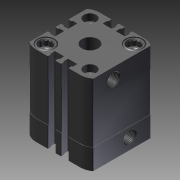
# Autodesk Inventor part: 536267 ADN-15-P---(Z)
Saved by Autodesk Inventor 2011 SP1 (Build 150282100, 282)
## iProperties
Created: 2018-05-26
Part Number: 536267 ADN-15-P---(Z)
Catalog Web Link: www.cadenas.de
Description: ADN-(Z)-Compact cylinder - Z
Vendor: FESTO
Document SubType Name: Modeling
Designer: psAdmin
Manufacturer: FESTO
Mass: 85.3695 g
Surface Area: 308.359 cm^2
Volume: 85.3695 cm^3
Density: 1 g/cm^3
Category: PARTsolutions
Company: FESTO
Title: 536267 ADN-15-P---(Z)
Author: Cadenas PARTsolutions
Comments: Compact cylinder - Z
PSOL_IDENT_0: {$CADENAS_DATA\23d-libs\festo\parts\a\adn\parts\adn_zr.prj},210 {VTYP=3D},{NB=536267 ADN-15-P---(Z)}
PSOL_IDENT_1: ,{LINA=536267 ADN-15-P---(Z)},{NN=ADN-(Z)},{DATE=06.10.2015 11:54:02},{GEOMDATE=22.09.2015 09:31:00}
PSOL_IDENT_2: ,{VERSION=},{LINEID=8220},{LINESUBID=-1},{WBVAR=HUB,DF,Q,S2S20,S1,R8,TT}  {NB=536267 ADN-15-P---(Z)}
PSOL_IDENT_3: ,{LINA=536267 ADN-15-P---(Z)},{KT=536267},{TNR=536267},{AUSF=ADN},{KDM=32},{BG=26.000},{VERS=2},{HUB
PSOL_IDENT_4: P=-},{HUB=15.00000},{HUB1=[1-400]},{HUB2=[1-300]},{HUB3=0},{THC='A','I'},{DF=P},{GA=A},{HUBL=variabl
PSOL_IDENT_5: e},{HUBC=hubc error},{Q=-},{VAR1C='-','Q'},{S2S20=-},{VAR2C='-','S2','S20'},{VAR5C='-','S6'},{S1=-},
PSOL_IDENT_6: {R8=-},{R81='-','R8'},{TT=-},{TT1='-','TT'},{VAR6C='-'},{VAR7C='-','R3'},{HUBALG=[1-400]},{A=19.000}
PSOL_IDENT_7: ,{A1=0.000},{AF=16.000},{AF1=0.000},{AF2=14.000},{AF3=0.000},{B=0.000},{B1=27.000},{BG1=0.000},{D1=9
PSOL_IDENT_8: .000},{D2=9.000},{D3=5.100},{D4=17.000},{D5=8.000},{D6=M5},{D7=5.000},{D8=4.500},{D9=8.000},{E=47.00
PSOL_IDENT_9: 0},{EE=G1/8},{EEN=9.728},{EE1=-},{J=15.000},{J1=6.000},{J11=6},{J2=0.000},{KF=5/16-24 UNF-2B},{KF1=-
PSOL_IDENT_10: },{KF2=10-32 UNF-2B},{KF3=-},{KK=3/8-24 UNF-2A},{KK1=-},{L1=3.300},{L2=44.000},{L3=2.100},{L4=5.000}
PSOL_IDENT_11: ,{L5=6.000},{L6=60.000},{L7=28.000},{L8=3.000},{L9=2.600},{L10=0.000},{L11=0.000},{MF=10.000},{MM=12
PSOL_IDENT_12: .000},{MM1=0.000},{PL=8.200},{RT=M6},{RTN=6},{RTNK=4.917},{SF=3/8},{SF1=-},{SW=10.000},{TG=32.500},{
PSOL_IDENT_13: VD=0.000},{VD1=6.400},{WH=6.200},{WH1=0.000},{WL=4.700},{WL1=0.000},{Y1=0.300},{Y2=0.500},{ZJ=50.200
PSOL_IDENT_14: },{ZM=56.400},{RU=35.200},{R1=12.400},{R2=1.000},{RA=9.700},{RB1=5.400},{RB2=6.800},{RT1=3.400},{DSK=
PSOL_IDENT_15: 9.000},{MDK=13.000},{MK=8.000},{MT=4.000},{MS=6.000},{RUB=0.600},{KFN=8.000},{KFK=6.647},{B111=12.80
PSOL_IDENT_16: 0},{B11=1.000},{B2=7.000},{B3=11.900},{B4=4.600},{B5=4.400},{B6=8.500},{B7=26.000},{B8=6.000},{B9=9.
PSOL_IDENT_17: 000},{B10=10.000},{W=0.400},{S=8.000},{LA=0.000},{LA1=0.000},{LA2=8.000},{LA3=12.500},{LA31=12.500},
PSOL_IDENT_18: {LA4=0.000},{LA5=0.000},{LA6=0.000},{RR=6.000},{LA7=0.000},{LA8=0.000},{LA9=0.000},{LA10=0.000},{ES=
PSOL_IDENT_19: 0.000},{SS=0.000},{TS=0.000},{WS=0.000},{DK=0.000},{KS=0.000},{QN=},{S2N=},{S1S20N=},{R8N=},{TTN=},{
PSOL_IDENT_20: DFALG='P','PPS'}
NN: ADN-(Z)
NT: Compact cylinder - Z
NB: 536267 ADN-15-P---(Z)
NBSYN: $TNR. $AUSF.-$HUB.-$DF.$QN.$S2N.$S1S20N.$R8N.$TTN.---(Z)
LINA: 536267 ADN-15-P---(Z)
TNR: 536267
AUSF: ADN
KDM: 32
BG: 26.000
HUB: 15.00000
DF: P
GA: A
Q: -
S2S20: -
S1: -
R8: -
TT: -
A: 19.000
A1: 0.000
AF: 16.000
AF1: 0.000
AF2: 14.000
AF3: 0.000
B: 0.000
B1: 27.000
BG1: 0.000
D1: 9.000
D2: 9.000
D3: 5.100
D4: 17.000
D5: 8.000
D6: M5
D7: 5.000
D8: 4.500
D9: 8.000
E: 47.000
EE: G1/8
EE1: -
J: 15.000
J1: 6.000
J2: 0.000
KF: 5/16-24 UNF-2B
KF1: -
KF2: 10-32 UNF-2B
KF3: -
KK: 3/8-24 UNF-2A
KK1: -
L1: 3.300
L2: 44.000
L3: 2.100
L4: 5.000
L5: 6.000
L6: 60.000
L7: 28.000
L8: 3.000
L9: 2.600
L10: 0.000
L11: 0.000
MF: 10.000
MM: 12.000
MM1: 0.000
PL: 8.200
RT: M6
RTNK: 4.917
SF: 3/8
SF1: -
SW: 10.000
TG: 32.500
VD: 0.000
VD1: 6.400
WH: 6.200
WH1: 0.000
WL: 4.700
WL1: 0.000
Y1: 0.300
Y2: 0.500
ZJ: 50.200
ZM: 56.400
RU: 35.200
R1: 12.400
R2: 1.000
RA: 9.700
DSK: 9.000
MDK: 13.000
MK: 8.000
MT: 4.000
MS: 6.000
RUB: 0.600
B111: 12.800
B11: 1.000
B2: 7.000
B3: 11.900
B4: 4.600
B5: 4.400
B6: 8.500
B7: 26.000
B8: 6.000
B9: 9.000
B10: 10.000
W: 0.400
S: 8.000
LA: 0.000
LA1: 0.000
LA2: 8.000
LA3: 12.500
LA31: 12.500
LA4: 0.000
LA5: 0.000
LA6: 0.000
RR: 6.000
LA7: 0.000
LA8: 0.000
LA9: 0.000
LA10: 0.000
ES: 0.000
SS: 0.000
TS: 0.000
WS: 0.000
DK: 0.000
KS: 0.000
SUPPLIER: FESTO
ARTICLENO: 536267 ADN-15-P---(Z)
BOMINFO: 536267 ADN-15-P---(Z)
CREATOR: CADENAS GmbH
Autodesk Inventor part; units mm, degrees
sketch "Skizze_2" plane through (0, 0, 0) normal (0, 0, 1) x (1, 0, 0)
  arc A0 (-23.5, -1.75) -> (-23.1, -2.15) centre (-23.1, -1.75) ccw
  line L0 (-23.1, -2.15) -> (-21.2, -2.15)
  arc A1 (-21.2, -2.15) -> (-21, -1.95) centre (-21.2, -1.95) ccw
  line L1 (-21, -1.95) -> (-21, -1.65)
  arc A2 (-20.8, -1.45) -> (-21, -1.65) centre (-20.8, -1.65) ccw
  line L2 (-20.8, -1.45) -> (-18, -1.45)
  arc A3 (-17.6, -1.85) -> (-18, -1.45) centre (-18, -1.85) ccw
  line L3 (-17.6, -1.85) -> (-17.6, -7.85)
  arc A4 (-18, -8.25) -> (-17.6, -7.85) centre (-18, -7.85) ccw
  line L4 (-18, -8.25) -> (-20.8, -8.25)
  arc A5 (-21, -8.05) -> (-20.8, -8.25) centre (-20.8, -8.05) ccw
  line L5 (-21, -8.05) -> (-21, -7.75)
  arc A6 (-21, -7.75) -> (-21.2, -7.55) centre (-21.2, -7.75) ccw
  line L6 (-21.2, -7.55) -> (-23.1, -7.55)
  arc A7 (-23.1, -7.55) -> (-23.5, -7.95) centre (-23.1, -7.95) ccw
  line L7 (-23.5, -7.95) -> (-23.5, -20.634)
  arc A8 (-23.5, -20.634) -> (-23.0482, -21.4703) centre (-22.5, -20.634) ccw
  arc A9 (-23.0482, -21.4703) -> (-16.25, -23.5) centre (-16.25, -11.1) ccw
  line L8 (-16.25, -23.5) -> (-7.95, -23.5)
  arc A10 (-7.95, -23.5) -> (-7.55, -23.1) centre (-7.95, -23.1) ccw
  line L9 (-7.55, -23.1) -> (-7.55, -21.2)
  arc A11 (-7.55, -21.2) -> (-7.75, -21) centre (-7.75, -21.2) ccw
  line L10 (-7.75, -21) -> (-8.05, -21)
  arc A12 (-8.25, -20.8) -> (-8.05, -21) centre (-8.05, -20.8) ccw
  line L11 (-8.25, -20.8) -> (-8.25, -18)
  arc A13 (-7.85, -17.6) -> (-8.25, -18) centre (-7.85, -18) ccw
  line L12 (-7.85, -17.6) -> (-1.85, -17.6)
  arc A14 (-1.45, -18) -> (-1.85, -17.6) centre (-1.85, -18) ccw
  line L13 (-1.45, -18) -> (-1.45, -20.8)
  arc A15 (-1.65, -21) -> (-1.45, -20.8) centre (-1.65, -20.8) ccw
  line L14 (-1.65, -21) -> (-1.95, -21)
  arc A16 (-1.95, -21) -> (-2.15, -21.2) centre (-1.95, -21.2) ccw
  line L15 (-2.15, -21.2) -> (-2.15, -23.1)
  arc A17 (-2.15, -23.1) -> (-1.75, -23.5) centre (-1.75, -23.1) ccw
  line L16 (-1.75, -23.5) -> (1.75, -23.5)
  arc A18 (1.75, -23.5) -> (2.15, -23.1) centre (1.75, -23.1) ccw
  line L17 (2.15, -23.1) -> (2.15, -21.2)
  arc A19 (2.15, -21.2) -> (1.95, -21) centre (1.95, -21.2) ccw
  line L18 (1.95, -21) -> (1.65, -21)
  arc A20 (1.45, -20.8) -> (1.65, -21) centre (1.65, -20.8) ccw
  line L19 (1.45, -20.8) -> (1.45, -18)
  arc A21 (1.85, -17.6) -> (1.45, -18) centre (1.85, -18) ccw
  line L20 (1.85, -17.6) -> (7.85, -17.6)
  arc A22 (8.25, -18) -> (7.85, -17.6) centre (7.85, -18) ccw
  line L21 (8.25, -18) -> (8.25, -20.8)
  arc A23 (8.05, -21) -> (8.25, -20.8) centre (8.05, -20.8) ccw
  line L22 (8.05, -21) -> (7.75, -21)
  arc A24 (7.75, -21) -> (7.55, -21.2) centre (7.75, -21.2) ccw
  line L23 (7.55, -21.2) -> (7.55, -23.1)
  arc A25 (7.55, -23.1) -> (7.95, -23.5) centre (7.95, -23.1) ccw
  line L24 (7.95, -23.5) -> (16.25, -23.5)
  arc A26 (16.25, -23.5) -> (23.0482, -21.4703) centre (16.25, -11.1) ccw
  arc A27 (23.0482, -21.4703) -> (23.5, -20.634) centre (22.5, -20.634) ccw
  line L25 (23.5, -20.634) -> (23.5, 20.634)
  arc A28 (23.5, 20.634) -> (23.0482, 21.4703) centre (22.5, 20.634) ccw
  arc A29 (23.0482, 21.4703) -> (16.25, 23.5) centre (16.25, 11.1) ccw
  line L26 (16.25, 23.5) -> (7.95, 23.5)
  arc A30 (7.95, 23.5) -> (7.55, 23.1) centre (7.95, 23.1) ccw
  line L27 (7.55, 23.1) -> (7.55, 21.2)
  arc A31 (7.55, 21.2) -> (7.75, 21) centre (7.75, 21.2) ccw
  line L28 (7.75, 21) -> (8.05, 21)
  arc A32 (8.25, 20.8) -> (8.05, 21) centre (8.05, 20.8) ccw
  line L29 (8.25, 20.8) -> (8.25, 18)
  arc A33 (7.85, 17.6) -> (8.25, 18) centre (7.85, 18) ccw
  line L30 (7.85, 17.6) -> (1.85, 17.6)
  arc A34 (1.45, 18) -> (1.85, 17.6) centre (1.85, 18) ccw
  line L31 (1.45, 18) -> (1.45, 20.8)
  arc A35 (1.65, 21) -> (1.45, 20.8) centre (1.65, 20.8) ccw
  line L32 (1.65, 21) -> (1.95, 21)
  arc A36 (1.95, 21) -> (2.15, 21.2) centre (1.95, 21.2) ccw
  line L33 (2.15, 21.2) -> (2.15, 23.1)
  arc A37 (2.15, 23.1) -> (1.75, 23.5) centre (1.75, 23.1) ccw
  line L34 (1.75, 23.5) -> (-1.75, 23.5)
  arc A38 (-1.75, 23.5) -> (-2.15, 23.1) centre (-1.75, 23.1) ccw
  line L35 (-2.15, 23.1) -> (-2.15, 21.2)
  arc A39 (-2.15, 21.2) -> (-1.95, 21) centre (-1.95, 21.2) ccw
  line L36 (-1.95, 21) -> (-1.65, 21)
  arc A40 (-1.45, 20.8) -> (-1.65, 21) centre (-1.65, 20.8) ccw
  line L37 (-1.45, 20.8) -> (-1.45, 18)
  arc A41 (-1.85, 17.6) -> (-1.45, 18) centre (-1.85, 18) ccw
  line L38 (-1.85, 17.6) -> (-7.85, 17.6)
  arc A42 (-8.25, 18) -> (-7.85, 17.6) centre (-7.85, 18) ccw
  line L39 (-8.25, 18) -> (-8.25, 20.8)
  arc A43 (-8.05, 21) -> (-8.25, 20.8) centre (-8.05, 20.8) ccw
  line L40 (-8.05, 21) -> (-7.75, 21)
  arc A44 (-7.75, 21) -> (-7.55, 21.2) centre (-7.75, 21.2) ccw
  line L41 (-7.55, 21.2) -> (-7.55, 23.1)
  arc A45 (-7.55, 23.1) -> (-7.95, 23.5) centre (-7.95, 23.1) ccw
  line L42 (-7.95, 23.5) -> (-16.25, 23.5)
  arc A46 (-16.25, 23.5) -> (-23.0482, 21.4703) centre (-16.25, 11.1) ccw
  arc A47 (-23.0482, 21.4703) -> (-23.5, 20.634) centre (-22.5, 20.634) ccw
  line L43 (-23.5, 20.634) -> (-23.5, 7.95)
  arc A48 (-23.5, 7.95) -> (-23.1, 7.55) centre (-23.1, 7.95) ccw
  line L44 (-23.1, 7.55) -> (-21.2, 7.55)
  arc A49 (-21.2, 7.55) -> (-21, 7.75) centre (-21.2, 7.75) ccw
  line L45 (-21, 7.75) -> (-21, 8.05)
  arc A50 (-20.8, 8.25) -> (-21, 8.05) centre (-20.8, 8.05) ccw
  line L46 (-20.8, 8.25) -> (-18, 8.25)
  arc A51 (-17.6, 7.85) -> (-18, 8.25) centre (-18, 7.85) ccw
  line L47 (-17.6, 7.85) -> (-17.6, 1.85)
  arc A52 (-18, 1.45) -> (-17.6, 1.85) centre (-18, 1.85) ccw
  line L48 (-18, 1.45) -> (-20.8, 1.45)
  arc A53 (-21, 1.65) -> (-20.8, 1.45) centre (-20.8, 1.65) ccw
  line L49 (-21, 1.65) -> (-21, 1.95)
  arc A54 (-21, 1.95) -> (-21.2, 2.15) centre (-21.2, 1.95) ccw
  line L50 (-21.2, 2.15) -> (-23.1, 2.15)
  arc A55 (-23.1, 2.15) -> (-23.5, 1.75) centre (-23.1, 1.75) ccw
  line L51 (-23.5, 1.75) -> (-23.5, -1.75)
  constraints: 112 point on circle, 104 end point, 56 centre point
extrude "Extrusion1" add sketch "Skizze_2" against normal blind 59
sketch "Sketch_113" plane through (0, 0, -15) normal (0, 0, 1) x (1, 0, 0)
  line L0 (-47, -47) -> (47, -47)
  line L1 (47, -47) -> (47, 47)
  line L2 (47, 47) -> (-47, 47)
  line L3 (-47, 47) -> (-47, -47)
  arc A0 (-23.25, -1.75) -> (-22.85, -2.15) centre (-22.85, -1.75) ccw
  line L4 (-22.85, -2.15) -> (-21, -2.15)
  line L5 (-21, -2.15) -> (-21, -7.55)
  line L6 (-21, -7.55) -> (-22.85, -7.55)
  arc A1 (-22.85, -7.55) -> (-23.25, -7.95) centre (-22.85, -7.95) ccw
  line L7 (-23.25, -7.95) -> (-23.25, -20.5433)
  arc A2 (-23.25, -20.5433) -> (-22.7763, -21.3936) centre (-22.25, -20.5433) ccw
  arc A3 (-22.7763, -21.3936) -> (-16.25, -23.25) centre (-16.25, -10.85) ccw
  line L8 (-16.25, -23.25) -> (-7.95, -23.25)
  arc A4 (-7.95, -23.25) -> (-7.55, -22.85) centre (-7.95, -22.85) ccw
  line L9 (-7.55, -22.85) -> (-7.55, -21)
  line L10 (-7.55, -21) -> (-2.15, -21)
  line L11 (-2.15, -21) -> (-2.15, -22.85)
  arc A5 (-2.15, -22.85) -> (-1.75, -23.25) centre (-1.75, -22.85) ccw
  line L12 (-1.75, -23.25) -> (1.75, -23.25)
  arc A6 (1.75, -23.25) -> (2.15, -22.85) centre (1.75, -22.85) ccw
  line L13 (2.15, -22.85) -> (2.15, -21)
  line L14 (2.15, -21) -> (7.55, -21)
  line L15 (7.55, -21) -> (7.55, -22.85)
  arc A7 (7.55, -22.85) -> (7.95, -23.25) centre (7.95, -22.85) ccw
  line L16 (7.95, -23.25) -> (16.25, -23.25)
  arc A8 (16.25, -23.25) -> (22.7763, -21.3936) centre (16.25, -10.85) ccw
  arc A9 (22.7763, -21.3936) -> (23.25, -20.5433) centre (22.25, -20.5433) ccw
  line L17 (23.25, -20.5433) -> (23.25, 20.5433)
  arc A10 (23.25, 20.5433) -> (22.7763, 21.3936) centre (22.25, 20.5433) ccw
  arc A11 (22.7763, 21.3936) -> (16.25, 23.25) centre (16.25, 10.85) ccw
  line L18 (16.25, 23.25) -> (7.95, 23.25)
  arc A12 (7.95, 23.25) -> (7.55, 22.85) centre (7.95, 22.85) ccw
  line L19 (7.55, 22.85) -> (7.55, 21)
  line L20 (7.55, 21) -> (2.15, 21)
  line L21 (2.15, 21) -> (2.15, 22.85)
  arc A13 (2.15, 22.85) -> (1.75, 23.25) centre (1.75, 22.85) ccw
  line L22 (1.75, 23.25) -> (-1.75, 23.25)
  arc A14 (-1.75, 23.25) -> (-2.15, 22.85) centre (-1.75, 22.85) ccw
  line L23 (-2.15, 22.85) -> (-2.15, 21)
  line L24 (-2.15, 21) -> (-7.55, 21)
  line L25 (-7.55, 21) -> (-7.55, 22.85)
  arc A15 (-7.55, 22.85) -> (-7.95, 23.25) centre (-7.95, 22.85) ccw
  line L26 (-7.95, 23.25) -> (-16.25, 23.25)
  arc A16 (-16.25, 23.25) -> (-22.7763, 21.3936) centre (-16.25, 10.85) ccw
  arc A17 (-22.7763, 21.3936) -> (-23.25, 20.5433) centre (-22.25, 20.5433) ccw
  line L27 (-23.25, 20.5433) -> (-23.25, 7.95)
  arc A18 (-23.25, 7.95) -> (-22.85, 7.55) centre (-22.85, 7.95) ccw
  line L28 (-22.85, 7.55) -> (-21, 7.55)
  line L29 (-21, 7.55) -> (-21, 2.15)
  line L30 (-21, 2.15) -> (-22.85, 2.15)
  arc A19 (-22.85, 2.15) -> (-23.25, 1.75) centre (-22.85, 1.75) ccw
  line L31 (-23.25, 1.75) -> (-23.25, -1.75)
  constraints: 64 end point, 40 point on circle, 20 centre point
extrude "Extrusion2" cut sketch "Sketch_113" against normal blind 29
sketch "Sketch_11_ALT_Drilling_1" plane through (0, -6, 0) normal (0, 1, 0) x (1, 0, 0)
  line L0 (23.5, 8.2) -> (11, 8.2)
  line L1 (11, 8.2) -> (11, 12.483)
  line L2 (11, 12.483) -> (22.919, 12.483)
  line L3 (22.919, 12.483) -> (23.5, 13.064)
  line L4 (23.5, 13.064) -> (23.5, 8.2)
  line L5 (23.5, 8.2) -> (11, 8.2)
  constraints: 12 end point
revolve "Revolution1" cut sketch "Sketch_11_ALT_Drilling_1" angle 360 about axis through (23.5, -6, -8.2) along (1, 0, 0)
thread "Thread1" size "G9.728x0.907" designation "G 1/8" standard "ISO Pipe Threads" length 7.419
sketch "Sketch_12_ALT_Drilling_2" plane through (0, 6, 0) normal (0, 1, 0) x (1, 0, 0)
  line L0 (23.5, 50.8) -> (11, 50.8)
  line L1 (11, 50.8) -> (11, 55.083)
  line L2 (11, 55.083) -> (22.919, 55.083)
  line L3 (22.919, 55.083) -> (23.5, 55.664)
  line L4 (23.5, 55.664) -> (23.5, 50.8)
  line L5 (23.5, 50.8) -> (11, 50.8)
  constraints: 12 end point
revolve "Revolution2" cut sketch "Sketch_12_ALT_Drilling_2" angle 360 about axis through (23.5, 6, -50.8) along (1, 0, 0)
thread "Thread2" size "G9.728x0.907" designation "G 1/8" standard "ISO Pipe Threads" length 7.419
sketch "Skizze_5_ALT_Drilling_3" plane through (0, 0, 0) normal (1, 0, 0) x (0, 1, 0)
  line L0 (0, -42.6) -> (0, 7.4)
  line L1 (0, 7.4) -> (6, 7.4)
  line L2 (6, 7.4) -> (6, -19.6)
  line L3 (6, -19.6) -> (16, -19.6)
  line L4 (16, -19.6) -> (16, -42.6)
  line L5 (16, -42.6) -> (0, -42.6)
  line L6 (0, -42.6) -> (0, 7.4)
  constraints: 14 end point
revolve "Revolution3" cut sketch "Skizze_5_ALT_Drilling_3" angle 360 about axis through (0, 0, -42.6) along (0, 0, -1)
sketch "Skizze_7_ALT_Drilling_4" plane through (0, 0, 0) normal (1, 0, 0) x (0, 1, 0)
  line L0 (0, -59) -> (0, -56.9)
  line L1 (0, -56.9) -> (4.5, -56.9)
  line L2 (4.5, -56.9) -> (4.5, -59)
  line L3 (4.5, -59) -> (0, -59)
  line L4 (0, -59) -> (0, -56.9)
  constraints: 10 end point
revolve "Revolution4" cut sketch "Skizze_7_ALT_Drilling_4" angle 360 about axis through (0, 0, -59) along (0, 0, -1)
sketch "Skizze_8_ALT_Drilling_5" plane through (16.25, 0, 0) normal (1, 0, 0) x (0, 0, -1)
  line L0 (26, 16.25) -> (0, 16.25)
  line L1 (0, 16.25) -> (0, 22.65)
  line L2 (0, 22.65) -> (7, 22.65)
  line L3 (7, 22.65) -> (7, 20.75)
  line L4 (7, 20.75) -> (26, 20.75)
  line L5 (26, 20.75) -> (26, 16.25)
  line L6 (26, 16.25) -> (0, 16.25)
  constraints: 14 end point
revolve "Revolution5" cut sketch "Skizze_8_ALT_Drilling_5" angle 360 about axis through (16.25, 16.25, -26) along (0, 0, -1)
sketch "Sketch_27" plane through (16.25, 0, 0) normal (1, 0, 0) x (0, 0, -1)
  line L0 (26, 16.25) -> (0, 16.25)
  line L1 (0, 21.25) -> (1.299, 20.5)
  line L2 (1.299, 20.5) -> (4.6, 20.5)
  line L3 (4.6, 20.5) -> (4.6, 19.25)
  line L4 (4.6, 19.25) -> (5.1415, 18.7085)
  line L5 (5.1415, 18.7085) -> (26, 18.7085)
  line L6 (26, 18.7085) -> (26, 21.75)
  line L7 (26, 21.75) -> (7, 21.75)
  line L8 (7, 21.75) -> (7, 22.2)
  line L9 (7, 22.2) -> (0.4, 22.2)
  line L10 (0.4, 22.2) -> (0, 21.8)
  line L11 (0, 21.8) -> (0, 21.25)
  constraints: 24 end point
revolve "Revolution6" add sketch "Sketch_27" angle 360 about axis through (16.25, 16.25, -26) along (0, 0, -1)
thread "Thread3" size "M6x1" class "6H" standard "ISO Metric profile" full length
sketch "Sketch_1_ALT_Drilling_6" plane through (16.25, 0, 0) normal (1, 0, 0) x (0, 0, -1)
  line L0 (59, -16.25) -> (33, -16.25)
  line L1 (33, -16.25) -> (33, -11.75)
  line L2 (33, -11.75) -> (52, -11.75)
  line L3 (52, -11.75) -> (52, -9.85)
  line L4 (52, -9.85) -> (59, -9.85)
  line L5 (59, -9.85) -> (59, -16.25)
  line L6 (59, -16.25) -> (33, -16.25)
  constraints: 14 end point
revolve "Revolution7" cut sketch "Sketch_1_ALT_Drilling_6" angle 360 about axis through (16.25, -16.25, -59) along (0, 0, -1)
sketch "Sketch_28" plane through (16.25, 0, 0) normal (1, 0, 0) x (0, 0, -1)
  line L0 (59, -16.25) -> (33, -16.25)
  line L1 (33, -10.75) -> (33, -13.7915)
  line L2 (33, -13.7915) -> (53.8585, -13.7915)
  line L3 (53.8585, -13.7915) -> (54.4, -13.25)
  line L4 (54.4, -13.25) -> (54.4, -12)
  line L5 (54.4, -12) -> (57.701, -12)
  line L6 (57.701, -12) -> (59, -11.25)
  line L7 (59, -11.25) -> (59, -10.7)
  line L8 (59, -10.7) -> (58.6, -10.3)
  line L9 (58.6, -10.3) -> (52, -10.3)
  line L10 (52, -10.3) -> (52, -10.75)
  line L11 (52, -10.75) -> (33, -10.75)
  constraints: 24 end point
revolve "Revolution8" add sketch "Sketch_28" angle 360 about axis through (16.25, -16.25, -59) along (0, 0, -1)
thread "Thread4" size "M6x1" class "6H" standard "ISO Metric profile" full length
sketch "Skizze_9_ALT_Drilling_7" plane through (-16.25, 0, 0) normal (1, 0, 0) x (0, 0, -1)
  line L0 (29.5, -16.25) -> (0, -16.25)
  line L1 (0, -16.25) -> (0, -9.85)
  line L2 (0, -9.85) -> (7, -9.85)
  line L3 (7, -9.85) -> (7, -11.75)
  line L4 (7, -11.75) -> (26, -11.75)
  line L5 (26, -11.75) -> (26, -16.25)
  line L6 (26, -16.25) -> (0, -16.25)
  constraints: 14 end point
revolve "Revolution9" cut sketch "Skizze_9_ALT_Drilling_7" angle 360 about axis through (-16.25, -16.25, -29.5) along (0, 0, -1)
sketch "Sketch_2_ALT_Drilling_8" plane through (-16.25, 0, 0) normal (1, 0, 0) x (0, 0, -1)
  line L0 (59, 16.25) -> (33, 16.25)
  line L1 (33, 16.25) -> (33, 20.75)
  line L2 (33, 20.75) -> (52, 20.75)
  line L3 (52, 20.75) -> (52, 22.65)
  line L4 (52, 22.65) -> (59, 22.65)
  line L5 (59, 22.65) -> (59, 16.25)
  line L6 (59, 16.25) -> (33, 16.25)
  constraints: 14 end point
revolve "Revolution10" cut sketch "Sketch_2_ALT_Drilling_8" angle 360 about axis through (-16.25, 16.25, -59) along (0, 0, -1)
sketch "Sketch_29" plane through (-16.25, 0, 0) normal (1, 0, 0) x (0, 0, -1)
  line L0 (26, -16.25) -> (0, -16.25)
  line L1 (0, -11.25) -> (1.299, -12)
  line L2 (1.299, -12) -> (4.6, -12)
  line L3 (4.6, -12) -> (4.6, -13.25)
  line L4 (4.6, -13.25) -> (5.1415, -13.7915)
  line L5 (5.1415, -13.7915) -> (26, -13.7915)
  line L6 (26, -13.7915) -> (26, -10.75)
  line L7 (26, -10.75) -> (7, -10.75)
  line L8 (7, -10.75) -> (7, -10.3)
  line L9 (7, -10.3) -> (0.4, -10.3)
  line L10 (0.4, -10.3) -> (0, -10.7)
  line L11 (0, -10.7) -> (0, -11.25)
  constraints: 24 end point
revolve "Revolution11" add sketch "Sketch_29" angle 360 about axis through (-16.25, -16.25, -26) along (0, 0, -1)
thread "Thread5" size "M6x1" class "6H" standard "ISO Metric profile" full length
sketch "Sketch_30" plane through (-16.25, 0, 0) normal (1, 0, 0) x (0, 0, -1)
  line L0 (59, 16.25) -> (33, 16.25)
  line L1 (33, 21.75) -> (33, 18.7085)
  line L2 (33, 18.7085) -> (53.8585, 18.7085)
  line L3 (53.8585, 18.7085) -> (54.4, 19.25)
  line L4 (54.4, 19.25) -> (54.4, 20.5)
  line L5 (54.4, 20.5) -> (57.701, 20.5)
  line L6 (57.701, 20.5) -> (59, 21.25)
  line L7 (59, 21.25) -> (59, 21.8)
  line L8 (59, 21.8) -> (58.6, 22.2)
  line L9 (58.6, 22.2) -> (52, 22.2)
  line L10 (52, 22.2) -> (52, 21.75)
  line L11 (52, 21.75) -> (33, 21.75)
  constraints: 24 end point
revolve "Revolution12" add sketch "Sketch_30" angle 360 about axis through (-16.25, 16.25, -59) along (0, 0, -1)
thread "Thread6" size "M6x1" class "6H" standard "ISO Metric profile" full length
sketch "Skizze_12_ALT_Drilling_9" plane through (16.25, 0, 0) normal (1, 0, 0) x (0, 0, -1)
  line L0 (33, -16.25) -> (-0.1, -16.25)
  line L1 (-0.1, -16.25) -> (-0.1, -11.75)
  line L2 (-0.1, -11.75) -> (5, -11.75)
  line L3 (5, -11.75) -> (5, -13.25)
  line L4 (5, -13.25) -> (5.5415, -13.7915)
  line L5 (5.5415, -13.7915) -> (33, -13.7915)
  line L6 (33, -13.7915) -> (33, -16.25)
  line L7 (33, -16.25) -> (-0.1, -16.25)
  constraints: 16 end point
revolve "Revolution13" cut sketch "Skizze_12_ALT_Drilling_9" angle 360 about axis through (16.25, -16.25, -33) along (0, 0, -1)
thread "Thread7" size "M6x1" class "6H" standard "ISO Metric profile" length 9.4585
sketch "Sketch_123" plane through (16.25, 0, 0) normal (1, 0, 0) x (0, 0, -1)
  line L0 (33, -16.25) -> (15, -16.25)
  line L1 (15, -16.25) -> (15, -11.25)
  line L2 (15, -11.25) -> (33, -11.25)
  line L3 (33, -11.25) -> (33, -16.25)
  line L4 (33, -16.25) -> (15, -16.25)
  constraints: 10 end point
revolve "Revolution14" add sketch "Sketch_123" angle 360 about axis through (16.25, -16.25, -33) along (0, 0, -1)
sketch "Sketch_124_ALT_Drilling_10" plane through (16.25, 0, 0) normal (1, 0, 0) x (0, 0, -1)
  line L0 (33, -16.25) -> (15, -16.25)
  line L1 (15, -16.25) -> (15, -13.25)
  line L2 (15, -13.25) -> (33, -13.25)
  line L3 (33, -13.25) -> (33, -16.25)
  line L4 (33, -16.25) -> (15, -16.25)
  constraints: 10 end point
revolve "Revolution15" cut sketch "Sketch_124_ALT_Drilling_10" angle 360 about axis through (16.25, -16.25, -33) along (0, 0, -1)
sketch "Sketch_3_ALT_Drilling_11" plane through (16.25, 0, 0) normal (1, 0, 0) x (0, 0, -1)
  line L0 (59.1, 16.25) -> (29.5, 16.25)
  line L1 (29.5, 16.25) -> (29.5, 18.7085)
  line L2 (29.5, 18.7085) -> (53.4585, 18.7085)
  line L3 (53.4585, 18.7085) -> (54, 19.25)
  line L4 (54, 19.25) -> (54, 20.75)
  line L5 (54, 20.75) -> (59.1, 20.75)
  line L6 (59.1, 20.75) -> (59.1, 16.25)
  line L7 (59.1, 16.25) -> (29.5, 16.25)
  constraints: 16 end point
revolve "Revolution16" cut sketch "Sketch_3_ALT_Drilling_11" angle 360 about axis through (16.25, 16.25, -59.1) along (0, 0, -1)
thread "Thread8" size "M6x1" class "6H" standard "ISO Metric profile" length 9.4585
sketch "Sketch_117" plane through (16.25, 0, 0) normal (1, 0, 0) x (0, 0, -1)
  line L0 (44, 16.25) -> (26, 16.25)
  line L1 (26, 16.25) -> (26, 21.25)
  line L2 (26, 21.25) -> (44, 21.25)
  line L3 (44, 21.25) -> (44, 16.25)
  line L4 (44, 16.25) -> (26, 16.25)
  constraints: 10 end point
revolve "Revolution17" add sketch "Sketch_117" angle 360 about axis through (16.25, 16.25, -44) along (0, 0, -1)
sketch "Sketch_119_ALT_Drilling_12" plane through (16.25, 0, 0) normal (1, 0, 0) x (0, 0, -1)
  line L0 (44, 16.25) -> (26, 16.25)
  line L1 (26, 16.25) -> (26, 19.25)
  line L2 (26, 19.25) -> (44, 19.25)
  line L3 (44, 19.25) -> (44, 16.25)
  line L4 (44, 16.25) -> (26, 16.25)
  constraints: 10 end point
revolve "Revolution18" cut sketch "Sketch_119_ALT_Drilling_12" angle 360 about axis through (16.25, 16.25, -44) along (0, 0, -1)
sketch "Skizze_13_ALT_Drilling_13" plane through (-16.25, 0, 0) normal (1, 0, 0) x (0, 0, -1)
  line L0 (33, 16.25) -> (-0.1, 16.25)
  line L1 (-0.1, 16.25) -> (-0.1, 20.75)
  line L2 (-0.1, 20.75) -> (5, 20.75)
  line L3 (5, 20.75) -> (5, 19.25)
  line L4 (5, 19.25) -> (5.5415, 18.7085)
  line L5 (5.5415, 18.7085) -> (33, 18.7085)
  line L6 (33, 18.7085) -> (33, 16.25)
  line L7 (33, 16.25) -> (-0.1, 16.25)
  constraints: 16 end point
revolve "Revolution19" cut sketch "Skizze_13_ALT_Drilling_13" angle 360 about axis through (-16.25, 16.25, -33) along (0, 0, -1)
thread "Thread9" size "M6x1" class "6H" standard "ISO Metric profile" length 9.4585
sketch "Sketch_121" plane through (-16.25, 0, 0) normal (1, 0, 0) x (0, 0, -1)
  line L0 (33, 16.25) -> (15, 16.25)
  line L1 (15, 16.25) -> (15, 21.25)
  line L2 (15, 21.25) -> (33, 21.25)
  line L3 (33, 21.25) -> (33, 16.25)
  line L4 (33, 16.25) -> (15, 16.25)
  constraints: 10 end point
revolve "Revolution20" add sketch "Sketch_121" angle 360 about axis through (-16.25, 16.25, -33) along (0, 0, -1)
sketch "Sketch_122_ALT_Drilling_14" plane through (-16.25, 0, 0) normal (1, 0, 0) x (0, 0, -1)
  line L0 (33, 16.25) -> (15, 16.25)
  line L1 (15, 16.25) -> (15, 19.25)
  line L2 (15, 19.25) -> (33, 19.25)
  line L3 (33, 19.25) -> (33, 16.25)
  line L4 (33, 16.25) -> (15, 16.25)
  constraints: 10 end point
revolve "Revolution21" cut sketch "Sketch_122_ALT_Drilling_14" angle 360 about axis through (-16.25, 16.25, -33) along (0, 0, -1)
sketch "Sketch_4_ALT_Drilling_15" plane through (-16.25, 0, 0) normal (1, 0, 0) x (0, 0, -1)
  line L0 (59.1, -16.25) -> (29.5, -16.25)
  line L1 (29.5, -16.25) -> (29.5, -13.7915)
  line L2 (29.5, -13.7915) -> (53.4585, -13.7915)
  line L3 (53.4585, -13.7915) -> (54, -13.25)
  line L4 (54, -13.25) -> (54, -11.75)
  line L5 (54, -11.75) -> (59.1, -11.75)
  line L6 (59.1, -11.75) -> (59.1, -16.25)
  line L7 (59.1, -16.25) -> (29.5, -16.25)
  constraints: 16 end point
revolve "Revolution22" cut sketch "Sketch_4_ALT_Drilling_15" angle 360 about axis through (-16.25, -16.25, -59.1) along (0, 0, -1)
thread "Thread10" size "M6x1" class "6H" standard "ISO Metric profile" length 9.4585
sketch "Sketch_118" plane through (-16.25, 0, 0) normal (1, 0, 0) x (0, 0, -1)
  line L0 (44, -16.25) -> (26, -16.25)
  line L1 (26, -16.25) -> (26, -11.25)
  line L2 (26, -11.25) -> (44, -11.25)
  line L3 (44, -11.25) -> (44, -16.25)
  line L4 (44, -16.25) -> (26, -16.25)
  constraints: 10 end point
revolve "Revolution23" add sketch "Sketch_118" angle 360 about axis through (-16.25, -16.25, -44) along (0, 0, -1)
sketch "Sketch_120_ALT_Drilling_16" plane through (-16.25, 0, 0) normal (1, 0, 0) x (0, 0, -1)
  line L0 (44, -16.25) -> (26, -16.25)
  line L1 (26, -16.25) -> (26, -13.25)
  line L2 (26, -13.25) -> (44, -13.25)
  line L3 (44, -13.25) -> (44, -16.25)
  line L4 (44, -16.25) -> (26, -16.25)
  constraints: 10 end point
revolve "Revolution24" cut sketch "Sketch_120_ALT_Drilling_16" angle 360 about axis through (-16.25, -16.25, -44) along (0, 0, -1)
sketch "Sketch_8" plane through (0, 0, 0) normal (0, 0, 1) x (1, 0, 0)
  line L0 (-20.8688, -16.25) -> (-20.25, -17.3218)
  line L1 (-20.25, -17.3218) -> (-20.25, -18.5594)
  line L2 (-20.25, -18.5594) -> (-19.1782, -19.1782)
  line L3 (-19.1782, -19.1782) -> (-18.5594, -20.25)
  line L4 (-18.5594, -20.25) -> (-17.3218, -20.25)
  line L5 (-17.3218, -20.25) -> (-16.25, -20.8688)
  line L6 (-16.25, -20.8688) -> (-15.1782, -20.25)
  line L7 (-15.1782, -20.25) -> (-13.9406, -20.25)
  line L8 (-13.9406, -20.25) -> (-13.3218, -19.1782)
  line L9 (-13.3218, -19.1782) -> (-12.25, -18.5594)
  line L10 (-12.25, -18.5594) -> (-12.25, -17.3218)
  line L11 (-12.25, -17.3218) -> (-11.6312, -16.25)
  line L12 (-11.6312, -16.25) -> (-12.25, -15.1782)
  line L13 (-12.25, -15.1782) -> (-12.25, -13.9406)
  line L14 (-12.25, -13.9406) -> (-13.3218, -13.3218)
  line L15 (-13.3218, -13.3218) -> (-13.9406, -12.25)
  line L16 (-13.9406, -12.25) -> (-15.1782, -12.25)
  line L17 (-15.1782, -12.25) -> (-16.25, -11.6312)
  line L18 (-16.25, -11.6312) -> (-17.3218, -12.25)
  line L19 (-17.3218, -12.25) -> (-18.5594, -12.25)
  line L20 (-18.5594, -12.25) -> (-19.1782, -13.3218)
  line L21 (-19.1782, -13.3218) -> (-20.25, -13.9406)
  line L22 (-20.25, -13.9406) -> (-20.25, -15.1782)
  line L23 (-20.25, -15.1782) -> (-20.8688, -16.25)
  constraints: 48 end point
extrude "Extrusion3" cut sketch "Sketch_8" against normal blind 4.4
sketch "Sketch_7" plane through (0, 0, 0) normal (0, 0, 1) x (1, 0, 0)
  line L0 (11.6312, 16.25) -> (12.25, 15.1782)
  line L1 (12.25, 15.1782) -> (12.25, 13.9406)
  line L2 (12.25, 13.9406) -> (13.3218, 13.3218)
  line L3 (13.3218, 13.3218) -> (13.9406, 12.25)
  line L4 (13.9406, 12.25) -> (15.1782, 12.25)
  line L5 (15.1782, 12.25) -> (16.25, 11.6312)
  line L6 (16.25, 11.6312) -> (17.3218, 12.25)
  line L7 (17.3218, 12.25) -> (18.5594, 12.25)
  line L8 (18.5594, 12.25) -> (19.1782, 13.3218)
  line L9 (19.1782, 13.3218) -> (20.25, 13.9406)
  line L10 (20.25, 13.9406) -> (20.25, 15.1782)
  line L11 (20.25, 15.1782) -> (20.8688, 16.25)
  line L12 (20.8688, 16.25) -> (20.25, 17.3218)
  line L13 (20.25, 17.3218) -> (20.25, 18.5594)
  line L14 (20.25, 18.5594) -> (19.1782, 19.1782)
  line L15 (19.1782, 19.1782) -> (18.5594, 20.25)
  line L16 (18.5594, 20.25) -> (17.3218, 20.25)
  line L17 (17.3218, 20.25) -> (16.25, 20.8688)
  line L18 (16.25, 20.8688) -> (15.1782, 20.25)
  line L19 (15.1782, 20.25) -> (13.9406, 20.25)
  line L20 (13.9406, 20.25) -> (13.3218, 19.1782)
  line L21 (13.3218, 19.1782) -> (12.25, 18.5594)
  line L22 (12.25, 18.5594) -> (12.25, 17.3218)
  line L23 (12.25, 17.3218) -> (11.6312, 16.25)
  constraints: 48 end point
extrude "Extrusion4" cut sketch "Sketch_7" against normal blind 4.4
sketch "Sketch_9" plane through (0, 0, -59) normal (0, 0, 1) x (1, 0, 0)
  line L0 (-20.8688, 16.25) -> (-20.25, 15.1782)
  line L1 (-20.25, 15.1782) -> (-20.25, 13.9406)
  line L2 (-20.25, 13.9406) -> (-19.1782, 13.3218)
  line L3 (-19.1782, 13.3218) -> (-18.5594, 12.25)
  line L4 (-18.5594, 12.25) -> (-17.3218, 12.25)
  line L5 (-17.3218, 12.25) -> (-16.25, 11.6312)
  line L6 (-16.25, 11.6312) -> (-15.1782, 12.25)
  line L7 (-15.1782, 12.25) -> (-13.9406, 12.25)
  line L8 (-13.9406, 12.25) -> (-13.3218, 13.3218)
  line L9 (-13.3218, 13.3218) -> (-12.25, 13.9406)
  line L10 (-12.25, 13.9406) -> (-12.25, 15.1782)
  line L11 (-12.25, 15.1782) -> (-11.6312, 16.25)
  line L12 (-11.6312, 16.25) -> (-12.25, 17.3218)
  line L13 (-12.25, 17.3218) -> (-12.25, 18.5594)
  line L14 (-12.25, 18.5594) -> (-13.3218, 19.1782)
  line L15 (-13.3218, 19.1782) -> (-13.9406, 20.25)
  line L16 (-13.9406, 20.25) -> (-15.1782, 20.25)
  line L17 (-15.1782, 20.25) -> (-16.25, 20.8688)
  line L18 (-16.25, 20.8688) -> (-17.3218, 20.25)
  line L19 (-17.3218, 20.25) -> (-18.5594, 20.25)
  line L20 (-18.5594, 20.25) -> (-19.1782, 19.1782)
  line L21 (-19.1782, 19.1782) -> (-20.25, 18.5594)
  line L22 (-20.25, 18.5594) -> (-20.25, 17.3218)
  line L23 (-20.25, 17.3218) -> (-20.8688, 16.25)
  constraints: 48 end point
extrude "Extrusion5" cut sketch "Sketch_9" along normal blind 4.4
sketch "Sketch_10" plane through (0, 0, -59) normal (0, 0, 1) x (1, 0, 0)
  line L0 (11.6312, -16.25) -> (12.25, -17.3218)
  line L1 (12.25, -17.3218) -> (12.25, -18.5594)
  line L2 (12.25, -18.5594) -> (13.3218, -19.1782)
  line L3 (13.3218, -19.1782) -> (13.9406, -20.25)
  line L4 (13.9406, -20.25) -> (15.1782, -20.25)
  line L5 (15.1782, -20.25) -> (16.25, -20.8688)
  line L6 (16.25, -20.8688) -> (17.3218, -20.25)
  line L7 (17.3218, -20.25) -> (18.5594, -20.25)
  line L8 (18.5594, -20.25) -> (19.1782, -19.1782)
  line L9 (19.1782, -19.1782) -> (20.25, -18.5594)
  line L10 (20.25, -18.5594) -> (20.25, -17.3218)
  line L11 (20.25, -17.3218) -> (20.8688, -16.25)
  line L12 (20.8688, -16.25) -> (20.25, -15.1782)
  line L13 (20.25, -15.1782) -> (20.25, -13.9406)
  line L14 (20.25, -13.9406) -> (19.1782, -13.3218)
  line L15 (19.1782, -13.3218) -> (18.5594, -12.25)
  line L16 (18.5594, -12.25) -> (17.3218, -12.25)
  line L17 (17.3218, -12.25) -> (16.25, -11.6312)
  line L18 (16.25, -11.6312) -> (15.1782, -12.25)
  line L19 (15.1782, -12.25) -> (13.9406, -12.25)
  line L20 (13.9406, -12.25) -> (13.3218, -13.3218)
  line L21 (13.3218, -13.3218) -> (12.25, -13.9406)
  line L22 (12.25, -13.9406) -> (12.25, -15.1782)
  line L23 (12.25, -15.1782) -> (11.6312, -16.25)
  constraints: 48 end point
extrude "Extrusion6" cut sketch "Sketch_10" along normal blind 4.4
ref_plane "CYLINDER_XY" through (0, 0, -42.6) normal (0, 0, 1) x (1, 0, 0)
ref_plane "CYLINDER_YZ" through (0, 0, -42.6) normal (1, 0, 0) x (0, 1, 0)
ref_plane "CYLINDER_ZX" through (0, 0, -42.6) normal (0, 1, 0) x (0, 0, 1)
ref_plane "FDT_FRONT_XY" through (0, 0, 0) normal (0, 0, 1) x (0, -1, 0)
ref_plane "FDT_FRONT_YZ" through (0, 0, 0) normal (0, -1, 0) x (1, 0, 0)
ref_plane "FDT_FRONT_ZX" through (0, 0, 0) normal (1, 0, 0) x (0, 0, 1)
ref_plane "FDT_QSFRONT_XY" through (23.5, -6, -8.2) normal (1, 0, 0) x (0, -1, 0)
ref_plane "FDT_QSFRONT_YZ" through (23.5, -6, -8.2) normal (0, -1, 0) x (0, 0, -1)
ref_plane "FDT_QSFRONT_ZX" through (23.5, -6, -8.2) normal (0, 0, -1) x (1, 0, 0)
ref_plane "FDT_QSREAR_XY" through (23.5, 6, -50.8) normal (1, 0, 0) x (0, -1, 0)
ref_plane "FDT_QSREAR_YZ" through (23.5, 6, -50.8) normal (0, -1, 0) x (0, 0, -1)
ref_plane "FDT_QSREAR_ZX" through (23.5, 6, -50.8) normal (0, 0, -1) x (1, 0, 0)
ref_plane "FDT_REAR_XY" through (0, 0, -59) normal (0, 0, 1) x (0, -1, 0)
ref_plane "FDT_REAR_YZ" through (0, 0, -59) normal (0, -1, 0) x (1, 0, 0)
ref_plane "FDT_REAR_ZX" through (0, 0, -59) normal (1, 0, 0) x (0, 0, 1)
ref_plane "FDT_SLOT3_XY" through (4.85, 17.6, -29.5) normal (0, 1, 0) x (1, 0, 0)
ref_plane "FDT_SLOT3_YZ" through (4.85, 17.6, -29.5) normal (1, 0, 0) x (0, 0, -1)
ref_plane "FDT_SLOT3_ZX" through (4.85, 17.6, -29.5) normal (0, 0, -1) x (0, 1, 0)
ref_plane "FDT_SLOT4_XY" through (-4.85, 17.6, -29.5) normal (0, 1, 0) x (1, 0, 0)
ref_plane "FDT_SLOT4_YZ" through (-4.85, 17.6, -29.5) normal (1, 0, 0) x (0, 0, -1)
ref_plane "FDT_SLOT4_ZX" through (-4.85, 17.6, -29.5) normal (0, 0, -1) x (0, 1, 0)
ref_plane "FDT_SLOT5_XY" through (-17.6, 4.85, -29.5) normal (-1, 0, 0) x (0, 1, 0)
ref_plane "FDT_SLOT5_YZ" through (-17.6, 4.85, -29.5) normal (0, 1, 0) x (0, 0, -1)
ref_plane "FDT_SLOT5_ZX" through (-17.6, 4.85, -29.5) normal (0, 0, -1) x (-1, 0, 0)
ref_plane "FDT_SLOT6_XY" through (-17.6, -4.85, -29.5) normal (-1, 0, 0) x (0, 1, 0)
ref_plane "FDT_SLOT6_YZ" through (-17.6, -4.85, -29.5) normal (0, 1, 0) x (0, 0, -1)
ref_plane "FDT_SLOT6_ZX" through (-17.6, -4.85, -29.5) normal (0, 0, -1) x (-1, 0, 0)
ref_plane "FDT_SLOT7_XY" through (-4.85, -17.6, -29.5) normal (0, -1, 0) x (-1, 0, 0)
ref_plane "FDT_SLOT7_YZ" through (-4.85, -17.6, -29.5) normal (-1, 0, 0) x (0, 0, -1)
ref_plane "FDT_SLOT7_ZX" through (-4.85, -17.6, -29.5) normal (0, 0, -1) x (0, -1, 0)
ref_plane "FDT_SLOT8_XY" through (4.85, -17.6, -29.5) normal (0, -1, 0) x (-1, 0, 0)
ref_plane "FDT_SLOT8_YZ" through (4.85, -17.6, -29.5) normal (-1, 0, 0) x (0, 0, -1)
ref_plane "FDT_SLOT8_ZX" through (4.85, -17.6, -29.5) normal (0, 0, -1) x (0, -1, 0)
ref_plane "TO_DUMMY_XY" through (0, 0, 0) normal (0, 0, 1) x (1, 0, 0)
ref_plane "TO_DUMMY_YZ" through (0, 0, 0) normal (1, 0, 0) x (0, 1, 0)
ref_plane "TO_DUMMY_ZX" through (0, 0, 0) normal (0, 1, 0) x (0, 0, 1)
body "Solid1"
